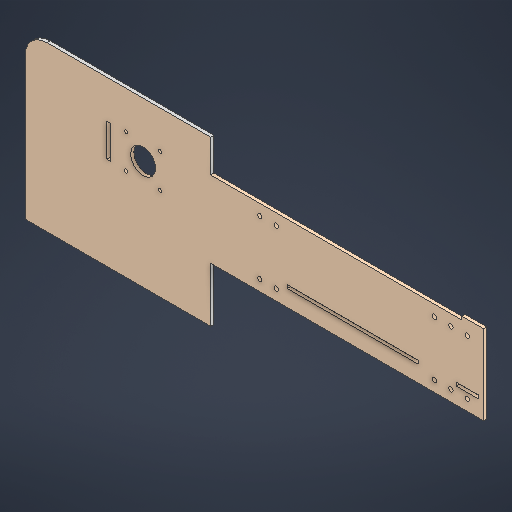
# Autodesk Inventor part: Sideboard
Saved by Autodesk Inventor 2027 (Build 310192000, 192)
## iProperties
Created: 2026-05-09
Part Number: Sideboard
Material: Generic
Document SubType Name: Modeling
Designer: alexy
Density: 1 g/cm^3
Appearance: Default
Author: alexy
Autodesk Inventor part; units mm, degrees
ref_plane "YZ Plane" through (0, 0, 0) normal (1, 0, 0) x (0, 1, 0)
ref_plane "XZ Plane" through (0, 0, 0) normal (0, 1, 0) x (-1, 0, 0)
ref_plane "XY Plane" through (0, 0, 0) normal (0, 0, 1) x (1, 0, 0)
sketch "Sketch1" plane through (0, 0, 0) normal (0, 0, 1) x (1, 0, 0)
  line L0 (0, 0) -> (350, 0)
  line L1 (350, 0) -> (350, 70)
  line L2 (350, 70) -> (0, 70)
  line L3 (0, 70) -> (0, 0)
  circle A0 centre (22.6, 65.5) radius 1.55
  circle A1 centre (22.6, 34.5) radius 1.55
  circle A2 centre (53.6, 65.5) radius 1.55
  circle A3 centre (53.6, 34.5) radius 1.55
  circle A4 centre (38.1, 50) radius 11.5
  line L4 (170, 18.1) -> (290, 18.1)
  line L5 (290, 18.1) -> (290, 15)
  line L6 (290, 15) -> (170, 15)
  line L7 (170, 15) -> (170, 18.1)
  line L8 (0, 70) -> (89.6145, 70)
  line L9 (250, 70) -> (287.051, 70)
  line L10 (250, 70) -> (270, 70)
  line L11 (270, 70) -> (270, 73)
  line L12 (270, 73) -> (250, 73)
  line L13 (250, 73) -> (250, 70)
  line L14 (310, 70) -> (310, 73)
  line L15 (310, 73) -> (290, 73)
  line L16 (290, 73) -> (290, 70)
  line L17 (290, 70) -> (327.051, 70)
  line L18 (290, 70) -> (310, 70)
  line L19 (350, 70) -> (350, 73)
  line L20 (350, 73) -> (330, 73)
  line L21 (330, 73) -> (330, 70)
  line L22 (330, 70) -> (367.051, 70)
  line L23 (330, 70) -> (350, 70)
  line L24 (8.1, 35) -> (5, 35)
  line L25 (5, 35) -> (5, 65)
  line L26 (5, 65) -> (8.1, 65)
  line L27 (8.1, 65) -> (8.1, 35)
  line L28 (8.1, 35) -> (5, 65) construction
  line L29 (5, 35) -> (8.1, 65) construction
  circle A5 centre (335, 10) radius 2.05
  circle A6 centre (320, 10) radius 2.05
  circle A7 centre (335, 60) radius 2.05
  circle A8 centre (320, 60) radius 2.05
  circle A9 centre (305, 60) radius 2.05
  circle A10 centre (305, 10) radius 2.05
  circle A11 centre (160, 10) radius 2.05
  circle A12 centre (145, 10) radius 2.05
  circle A13 centre (160, 60) radius 2.05
  circle A14 centre (145, 60) radius 2.05
  line L30 (325, 18.1) -> (345, 18.1)
  line L31 (345, 18.1) -> (345, 15)
  line L32 (345, 15) -> (325, 15)
  line L33 (325, 15) -> (325, 18.1)
  line L34 (0, 70) -> (100, 70)
  line L35 (100, 70) -> (100, 100)
  line L36 (100, 100) -> (0, 100)
  line L37 (0, 100) -> (0, 70)
  point P0 (6.55, 50)
  point P1 (5, 50)
  point P2 (8.1, 50)
  point P3 (170, 16.55)
  point P4 (290, 70)
  point P5 (100, 70)
  dimension "d1" = 3.1
  dimension "d2" = 3.1
  dimension "d3" = 3.1
  dimension "d4" = 3.1
  dimension "d5" = 31
  dimension "d7" = 23
  dimension "d8" = 15.5
  dimension "d9" = 15.5
  dimension "d10" = 70
  dimension "d11" = 31
  dimension "d12" = 3.1
  dimension "d13" = 50
  dimension "d46" = 20
  dimension "d47" = 3
  dimension "d48" = 20
  dimension "d49" = 3
  dimension "d50" = 20
  dimension "d51" = 3
  dimension "d52" = 20
  dimension "d53" = 20
  dimension "d54" = 350
  dimension "d55" = 3.1
  dimension "d56" = 5
  dimension "d57" = 15
  dimension "d58" = 30
  dimension "d59" = 120
  dimension "d63" = 4.1
  dimension "d64" = 4.1
  dimension "d65" = 4.1
  dimension "d66" = 4.1
  dimension "d67" = 4.1
  dimension "d68" = 4.1
  dimension "d69" = 15
  dimension "d70" = 15
  dimension "d71" = 10
  dimension "d72" = 10
  dimension "d73" = 15
  dimension "d79" = 4.1
  dimension "d80" = 4.1
  dimension "d81" = 4.1
  dimension "d82" = 4.1
  dimension "d85" = 15
  dimension "d87" = 10
  dimension "d88" = 10
  dimension "d89" = 10
  dimension "d90" = 60
  dimension "d91" = 5
  dimension "d92" = 20
  dimension "d93" = 15
  dimension "d94" = 100
  dimension "d95" = 30
  constraints: 76 end point, 16 parallel, 15 centre point, 13 horizontal alignment, 11 horizontal, 8 perpendicular, 8 vertical alignment, 5 midpoint, 1 coincident
  measures "d1" diameter of A0
  measures "d2" diameter of A1
  measures "d3" diameter of A2
  measures "d4" diameter of A3
  measures "d5" distance of A1.centre A3.centre
  measures "d7" diameter of A4
  measures "d8" horizontal distance of A0.centre A4.centre
  measures "d9" horizontal distance of A4.centre A3.centre
  measures "d10" distance of L0.end L1.end
  measures "d11" distance of A3.centre A2.centre
  measures "d12" distance of L6.end L4.start
  measures "d13" distance from line of L0 A4.centre
  measures "d46" distance of L12.end L12.start
  measures "d47" distance of L12.end L10.start
  measures "d48" distance of L16.start L14.end
  measures "d49" distance of L16.start L16.end
  measures "d50" distance of L21.start L19.end
  measures "d51" distance of L21.start L22.start
  measures "d52" distance of L16.start L12.start
  measures "d53" distance of L14.end L21.start
  measures "d54" distance of L0.end L0.start
  measures "d55" distance of L25.end L26.end
  measures "d56" distance between parallel lines of L3 L25
  measures "d57" distance of point (5, 50) L25.end
  measures "d58" distance of point (8.1, 50) A4.centre
  measures "d59" distance of L5.end L6.end
  measures "d63" diameter of A5
  measures "d64" diameter of A6
  measures "d65" diameter of A7
  measures "d66" diameter of A8
  measures "d67" diameter of A9
  measures "d68" diameter of A10
  measures "d69" distance of A6.centre A5.centre
  measures "d70" distance of A10.centre A6.centre
  measures "d71" distance from line of L0 A5.centre
  measures "d72" distance from line of L2 A7.centre
  measures "d73" distance from line of L1 A5.centre
  measures "d79" diameter of A11
  measures "d80" diameter of A12
  measures "d81" diameter of A13
  measures "d82" diameter of A14
  measures "d85" distance of A12.centre A11.centre
  measures "d87" horizontal distance of A11.centre L6.end
  measures "d88" distance from line of L0 A11.centre
  measures "d89" distance from line of L2 A13.centre
  measures "d90" distance between parallel lines of L1 L5
  measures "d91" distance between parallel lines of L1 L31
  measures "d92" distance between parallel lines of L31 L33
  measures "d93" distance between parallel lines of L0 L6
  measures "d94" distance of L36.end L35.end
  measures "d95" distance of L34.end L35.end
extrude "Extrusion1" add sketch "Sketch1" along normal blind 3 contours L3 L2 L1 L0 | L37 L36 L35 L2 | L2 L21 L20 L19
sketch "Sketch3" plane through (0, 0, 3) normal (0, 0, 1) x (1, 0, 0)
  line L0 (0, 100) -> (0, 0) projected
  line L1 (0, 100) -> (-70, 100)
  line L2 (-70, 100) -> (-70, -50)
  line L3 (-70, -50) -> (100, -50)
  line L4 (100, -50) -> (100, 0)
  line L5 (0, 0) -> (350, 0) projected
  dimension "d99" = 70
  dimension "d100" = 150
  dimension "d101" = 170
  constraints: 8 end point, 3 perpendicular, 1 horizontal, 1 point on line
  measures "d99" distance of L0.start L1.end
  measures "d100" distance of L1.end L2.end
  measures "d101" distance of L2.end L3.end
extrude "Extrusion3" add sketch "Sketch3" against normal blind 3
fillet "Fillet1" radius 20 1 edges at (-70, 100, 1.5)
body "Solid1"
